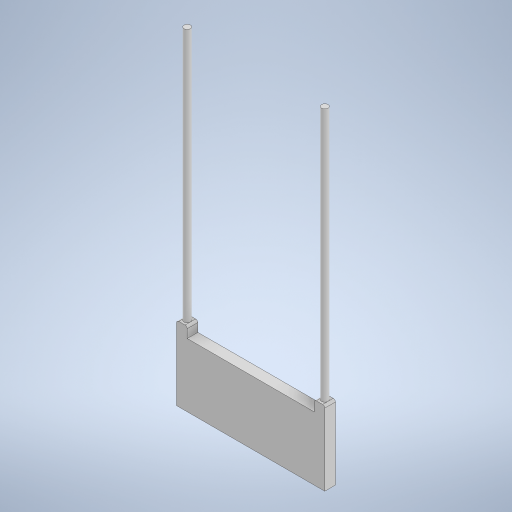
# Autodesk Inventor part: K71-6
Saved by Autodesk Inventor 2023 (Build 270158000, 158)
## iProperties
Created: 2023-12-13
Part Number: K71-6
Material: Generic
Document SubType Name: Sheet Metal
Designer: dank1
Density: 1 g/cm^3
Sheet Metal Rule: Default
Appearance: Default
Author: dank1
Autodesk Inventor part; units mm, degrees
ref_plane "YZ Plane" through (0, 0, 0) normal (1, 0, 0) x (0, 1, 0)
ref_plane "XZ Plane" through (0, 0, 0) normal (0, 1, 0) x (-1, 0, 0)
ref_plane "XY Plane" through (0, 0, 0) normal (0, 0, 1) x (1, 0, 0)
sketch "Sketch2" plane through (0, 0, 0) normal (0, 0, 1) x (1, 0, 0)
  line L0 (7, -3) -> (7, 3)
  line L1 (7, -3) -> (-7, -3)
  line L2 (-7, -3) -> (-7, 3)
  line L3 (6, 3) -> (6, 3.8)
  line L4 (6.2, 4) -> (6.8, 4)
  line L5 (7, 3.8) -> (7, 3)
  line L6 (-6, 3) -> (-6, 3.8)
  line L7 (-6.2, 4) -> (-6.8, 4)
  line L8 (-7, 3.8) -> (-7, 3)
  line L9 (-6, 3) -> (6, 3)
  line L10 (7, 3) -> (7.3028, 3)
  line L11 (-7, 3) -> (-7.3058, 3)
  arc A0 (-6, 3.8) -> (-6.2, 4) centre (-6.2, 3.8) ccw
  arc A1 (-6.8, 4) -> (-7, 3.8) centre (-6.8, 3.8) ccw
  arc A2 (6.2, 4) -> (6, 3.8) centre (6.2, 3.8) ccw
  arc A3 (7, 3.8) -> (6.8, 4) centre (6.8, 3.8) ccw
  point P0 (0, 0)
  dimension "d5" = 14
  dimension "d6" = 6
  constraints: 24 end point, 8 point on circle, 8 tangent, 4 centre point, 4 horizontal, 3 equal radius, 2 parallel, 1 vertical
  measures "d5" distance of L1.start L1.end
  measures "d6" distance of L1.start L0.end
extrude "Extrusion1" add sketch "Sketch2" along normal blind 1
sketch "Sketch3" plane through (-6.8, 4, 0) normal (0, 1, 0) x (1, 0, 0)
  circle A0 centre (0.3, -0.5) radius 0.3
  point P0 (6.8, 0)
  dimension "d9" = 0.6
  constraints: 1 centre point
  measures "d9" diameter of A0
sketch "Sketch4" plane through (6.2, 4, 0) normal (0, 1, 0) x (1, 0, 0)
  circle A0 centre (0.3, -0.5) radius 0.3
  point P0 (-6.2, 0)
  dimension "d10" = 0.6
  constraints: 1 centre point
  measures "d10" diameter of A0
extrude "Extrusion2" add sketch "Sketch4" along normal blind 24
extrude "Extrusion3" add sketch "Sketch3" along normal blind 24
equation "\"BendRadius\" = Thickness"
equation "\"BendReliefWidth\" = Thickness"
equation "\"BendReliefDepth\" = 0.5 * Thickness"
equation "\"CornerReliefSize\" = 4 * Thickness"
equation "\"MinimumRemnant\" = 2 * Thickness"
equation "\"TransitionRadius\" = BendRadius"
equation "\"JacobiRadiusSize\" = BendRadius"
equation "\"GapSize\" = Thickness"
equation "\"Thickness\" = 3.048"
body "Solid1"
